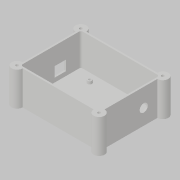
# Autodesk Inventor part: Pulsar_Box
Saved by Autodesk Inventor 2017.3 (Build 213256000, 256)
## iProperties
Created: 2018-02-02
Part Number: Pulsar_Box
Material: Generic
Document SubType Name: Modeling
Designer: Alex
Density: 1 g/cm^3
Appearance: Default
Author: Alex
Autodesk Inventor part; units mm, degrees
ref_plane "YZ Plane" through (0, 0, 0) normal (1, 0, 0) x (0, 1, 0)
ref_plane "XZ Plane" through (0, 0, 0) normal (0, 1, 0) x (-1, 0, 0)
ref_plane "XY Plane" through (0, 0, 0) normal (0, 0, 1) x (1, 0, 0)
sketch "Sketch1" plane through (0, 0, 0) normal (0, 1, 0) x (-1, 0, 0)
  line L0 (-45, 35) -> (-39, 35) construction
  line L1 (45, 35) -> (45, 29) construction
  line L2 (45, -35) -> (39, -35) construction
  line L3 (-45, -35) -> (-45, -29) construction
  line L4 (-45, 35) -> (45, -35) construction
  line L5 (45, 35) -> (-45, -35) construction
  arc A0 (40.2639, -31.3164) -> (39, -35) centre (45, -35) ccw construction
  arc A1 (-45, -29) -> (-39, -35) centre (-45, -35) ccw
  arc A2 (-40.2639, 31.3164) -> (-39, 35) centre (-45, 35) ccw construction
  arc A3 (45, 29) -> (39, 35) centre (45, 35) ccw
  line L6 (39, -35) -> (-39, -35)
  line L7 (45, -29) -> (45, -35) construction
  arc A4 (45, -29) -> (40.2639, -31.3164) centre (45, -35) ccw construction
  arc A5 (39, -35) -> (45, -29) centre (45, -35) ccw
  arc A6 (40.2639, 31.3164) -> (45, 29) centre (45, 35) ccw construction
  arc A7 (39, 35) -> (40.2639, 31.3164) centre (45, 35) ccw construction
  line L8 (39, 35) -> (45, 35) construction
  line L9 (45, 29) -> (45, -29)
  line L10 (-39, 35) -> (39, 35)
  line L11 (-45, 29) -> (-45, 35) construction
  arc A8 (-45, 29) -> (-40.2639, 31.3164) centre (-45, 35) ccw construction
  arc A9 (-39, 35) -> (-45, 29) centre (-45, 35) ccw
  arc A10 (-40.2639, -31.3164) -> (-45, -29) centre (-45, -35) ccw construction
  arc A11 (-39, -35) -> (-40.2639, -31.3164) centre (-45, -35) ccw construction
  line L12 (-39, -35) -> (-45, -35) construction
  line L13 (-45, -29) -> (-45, 29)
  point P0 (0, 0)
  dimension "d0" = 90
  dimension "d1" = 70
  dimension "d2" = 12
  constraints: 28 end point, 24 point on circle, 18 parallel, 12 centre point, 9 perpendicular, 4 coincident, 4 point on line, 3 equal radius, 3 horizontal, 2 midpoint
  measures "d0" distance of L2.start L3.start
  measures "d1" distance of L3.start L0.start
  measures "d2" diameter of A0
extrude "Extrusion1" add sketch "Sketch1" along normal blind 2
sketch "Sketch2" plane through (0, 2, 0) normal (0, 1, 0) x (1, 0, 0)
  line L0 (39, 35) -> (-39, 35) projected
  arc A0 (-39, 35) -> (-45, 29) centre (-45, 35) ccw projected
  line L1 (-45, 29) -> (-45, -29) projected
  arc A1 (-45, -29) -> (-39, -35) centre (-45, -35) ccw projected
  line L2 (-39, -35) -> (39, -35) projected
  arc A2 (39, -35) -> (45, -29) centre (45, -35) ccw projected
  line L3 (45, -29) -> (45, 29) projected
  arc A3 (45, 29) -> (39, 35) centre (45, 35) ccw projected
  line L4 (-41, 33) -> (41, 33)
  arc A4 (43, 31.5359) -> (41.5359, 33) centre (45, 35) ccw construction
  line L5 (43, 31) -> (43, -31)
  arc A5 (48.4641, -33) -> (43, -38.4641) centre (45, -35) ccw construction
  line L6 (41, -33) -> (-41, -33)
  arc A6 (-43, -31.5359) -> (-41.5359, -33) centre (-45, -35) ccw construction
  line L7 (-43, -31) -> (-43, 31)
  arc A7 (-48.4641, 33) -> (-43, 38.4641) centre (-45, 35) ccw construction
  arc A8 (-41, 33) -> (-43, 31) centre (-41, 31) ccw
  arc A9 (-43, -31) -> (-41, -33) centre (-41, -31) ccw
  arc A10 (41, -33) -> (43, -31) centre (41, -31) ccw
  arc A11 (43, 31) -> (41, 33) centre (41, 31) ccw
  point P0 (0, 0)
  dimension "d5" = 2
  dimension "d6" = 2
  constraints: 16 point on circle, 8 centre point, 8 end point, 8 point on line, 8 tangent, 3 equal radius, 7 other
  measures "d5" distance between parallel lines of L0 L4
  measures "d6" radius of A8
extrude "Extrusion2" add sketch "Sketch2" along normal blind 35
sketch "Sketch3" plane through (0, 2, 0) normal (0, 1, 0) x (1, 0, 0)
  arc A0 (-41, 33) -> (-43, 31) centre (-41, 31) ccw construction
  line L0 (-43, 31) -> (-43, -31) construction
  arc A1 (-43, -31) -> (-41, -33) centre (-41, -31) ccw construction
  line L1 (-41, -33) -> (41, -33) construction
  arc A2 (41, -33) -> (43, -31) centre (41, -31) ccw construction
  line L2 (43, -31) -> (43, 31) construction
  arc A3 (43, 31) -> (41, 33) centre (41, 31) ccw construction
  line L3 (41, 33) -> (-41, 33) construction
  arc A4 (-41, 33) -> (-43, 31) centre (-41, 31) ccw construction
  line L4 (-41, 33) -> (41, 33) construction
  arc A5 (43, 31) -> (41, 33) centre (41, 31) ccw construction
  line L5 (43, 31) -> (43, -31) construction
  arc A6 (41, -33) -> (43, -31) centre (41, -31) ccw construction
  line L6 (41, -33) -> (-41, -33) construction
  arc A7 (-43, -31) -> (-41, -33) centre (-41, -31) ccw construction
  line L7 (-43, -31) -> (-43, 31) construction
  line L8 (39, 35) -> (-39, 35) construction
  arc A8 (-39, 35) -> (-45, 29) centre (-45, 35) ccw construction
  line L9 (-45, 29) -> (-45, -29) construction
  arc A9 (-45, -29) -> (-39, -35) centre (-45, -35) ccw construction
  line L10 (-39, -35) -> (39, -35) construction
  arc A10 (39, -35) -> (45, -29) centre (45, -35) ccw construction
  line L11 (45, -29) -> (45, 29) construction
  arc A11 (45, 29) -> (39, 35) centre (45, 35) ccw construction
  circle A12 centre (-23.7, 23.4) radius 2.5
  circle A13 centre (27.1, 8.2) radius 2.5
  circle A14 centre (-25, -24.8) radius 2.5
  circle A15 centre (27.1, -19.7) radius 2.5
  line L12 (29.6, -27.3) -> (-39, -27.3) construction
  line L13 (-39, -27.3) -> (-39, 26) construction
  line L14 (-39, 26) -> (29.6, 26) construction
  line L15 (29.6, 26) -> (29.6, -27.3) construction
  line L16 (29.6, -27.3) -> (-39, 26) construction
  line L17 (-39, -27.3) -> (29.6, 26) construction
  circle A16 centre (-23.7, 23.4) radius 1.25
  circle A17 centre (27.1, 8.2) radius 1.25
  circle A18 centre (27.1, -19.7) radius 1.25
  circle A19 centre (-25, -24.8) radius 1.25
  point P0 (0, 0)
  point P1 (-4.7, -0.65)
  dimension "d9" = 5
  dimension "d10" = 53.3
  dimension "d11" = 68.6
  dimension "d12" = 2.5
  dimension "d13" = 5.1
  dimension "d14" = 27.9
  dimension "d15" = 15.2
  dimension "d16" = 14
  dimension "d17" = 1.3
  dimension "d18" = 50.8
  dimension "d19" = 4
  dimension "d20" = 7
  dimension "d21" = 2.5
  constraints: 12 end point, 8 centre point, 6 equal radius, 4 coincident, 2 midpoint, 2 parallel, 1 horizontal, 1 perpendicular, 1 vertical alignment
  measures "d9" diameter of A12
  measures "d10" distance of L12.end L13.end
  measures "d11" distance of L12.start L12.end
  measures "d12" distance from line of A14.centre L12
  measures "d13" vertical distance of A15.centre A14.centre
  measures "d14" distance of A13.centre A15.centre
  measures "d15" vertical distance of A12.centre A13.centre
  measures "d16" distance from line of L13 A14.centre
  measures "d17" horizontal distance of A12.centre A14.centre
  measures "d18" horizontal distance of A13.centre A12.centre
  measures "d19" distance between parallel lines of L0 L13
  measures "d20" distance between parallel lines of L4 L14
  measures "d21" diameter of A16
extrude "Extrusion3" add sketch "Sketch3" along normal blind 3
sketch "Sketch4" plane through (-43, 2, 31) normal (1, 0, 0) x (0, 0, -1)
  line L0 (62, 0) -> (0, 0) construction
  line L1 (62, 0) -> (62, 35) construction
  line L2 (0, 35) -> (62, 35) construction
  line L3 (0, 0) -> (0, 35) construction
  line L4 (2, -2) -> (60, -2) construction
  line L5 (2, -2) -> (2, 35) construction
  line L6 (60, 35) -> (2, 35) construction
  line L7 (60, -2) -> (60, 35) construction
  line L8 (8.7, 3) -> (3.7, 3) construction
  line L9 (3.7, 0) -> (8.7, 0) construction
  line L10 (3.7, 0) -> (3.7, 3) construction
  line L11 (8.7, 0) -> (8.7, 3) construction
  line L12 (4.95, 3) -> (7.45, 3) construction
  line L13 (7.45, 0) -> (4.95, 0) construction
  line L14 (4.95, 3) -> (7.45, 3) construction
  line L15 (7.45, 0) -> (7.45, 3) construction
  line L16 (4.95, 0) -> (4.95, 3) construction
  line L17 (56.9, 3) -> (51.9, 3) construction
  line L18 (51.9, 0) -> (56.9, 0) construction
  line L19 (56.9, 0) -> (56.9, 3) construction
  line L20 (51.9, 0) -> (51.9, 3) construction
  line L21 (53.15, 3) -> (55.65, 3) construction
  line L22 (53.15, 0) -> (53.15, 3) construction
  line L23 (55.65, 0) -> (55.65, 3) construction
  line L24 (0, 35) -> (62, 35) construction
  line L25 (47.7, 35) -> (47.7, 0) construction
  line L26 (62, 0) -> (0, 0) construction
  line L27 (35.2, 0) -> (35.2, 35) construction
  line L28 (54.4, -0.499) -> (54.4, 3) construction
  line L29 (35.2, 15.6) -> (47.7, 15.6)
  line L30 (47.7, 15.6) -> (47.7, 4.6)
  line L31 (47.7, 4.6) -> (35.2, 4.6)
  line L32 (35.2, 4.6) -> (35.2, 15.6)
  point P0 (31, -2)
  dimension "d25" = 6.7
  dimension "d26" = 12.5
  dimension "d27" = 11
  dimension "d28" = 1.6
  constraints: 14 end point, 4 point on line, 3 perpendicular, 2 parallel, 1 horizontal, 1 midpoint, 4 other
  measures "d25" distance between parallel lines of L25 L28
  measures "d26" distance between parallel lines of L27 L25
  measures "d27" distance between parallel lines of L31 L29
  measures "d28" distance between parallel lines of L31 L21
extrude "Extrusion4" cut sketch "Sketch4" against normal blind 3
sketch "Sketch5" plane through (45, 0, 29) normal (1, 0, 0) x (0, 0, -1)
  line L0 (58, 0) -> (0, 0) construction
  line L1 (58, 0) -> (58, 37) construction
  line L2 (0, 37) -> (58, 37) construction
  line L3 (0, 0) -> (0, 37) construction
  line L4 (33.2, 6.6) -> (33.2, 17.6) construction
  line L5 (33.2, 17.6) -> (45.7, 17.6) construction
  line L6 (45.7, 17.6) -> (45.7, 6.6) construction
  line L7 (45.7, 6.6) -> (33.2, 6.6) construction
  line L8 (60, 2) -> (-2, 2) construction
  line L9 (60, 2) -> (60, 37) construction
  line L10 (-2, 37) -> (60, 37) construction
  line L11 (-2, 2) -> (-2, 37) construction
  line L12 (33.2, 17.6) -> (45.7, 17.6) construction
  circle A0 centre (43, 17) radius 4.5
  line L13 (-2, 2) -> (60, 2) projected
  point P0 (29, 0)
  dimension "d31" = 9
  dimension "d32" = 15
  dimension "d33" = 15
  constraints: 1 centre point
  measures "d31" diameter of A0
  measures "d32" distance from line of L13 A0.centre
  measures "d33" distance from line of L1 A0.centre
extrude "Extrusion5" cut sketch "Sketch5" against normal blind 3
sketch "Sketch6" plane through (0, 37, 0) normal (0, 1, 0) x (1, 0, 0)
  arc A0 (-41, 33) -> (-43, 31) centre (-41, 31) ccw construction
  line L0 (-41, 33) -> (41, 33) construction
  arc A1 (43, 31) -> (41, 33) centre (41, 31) ccw construction
  line L1 (43, 31) -> (43, -31) construction
  arc A2 (41, -33) -> (43, -31) centre (41, -31) ccw construction
  line L2 (41, -33) -> (-41, -33) construction
  arc A3 (-43, -31) -> (-41, -33) centre (-41, -31) ccw construction
  line L3 (-43, -31) -> (-43, 31) construction
  line L4 (39, 35) -> (-39, 35) construction
  arc A4 (-39, 35) -> (-45, 29) centre (-45, 35) ccw construction
  line L5 (-45, 29) -> (-45, -29) construction
  arc A5 (-45, -29) -> (-39, -35) centre (-45, -35) ccw construction
  line L6 (-39, -35) -> (39, -35) construction
  arc A6 (39, -35) -> (45, -29) centre (45, -35) ccw construction
  line L7 (45, -29) -> (45, 29) construction
  arc A7 (45, 29) -> (39, 35) centre (45, 35) ccw construction
  arc A8 (39, -35) -> (45, -29) centre (45, -35) ccw projected
  point P0 (0, 0)
  constraints: 4 coincident
hole "Hole1" at (-45, 37, 35) at (-45, 37, -35) at (45, 37, -35) at (45, 37, 35) direction (0, -1, 0) diameter 3 depth 8 tip angle 118
sketch "Sketch7" plane through (39, 0, -35) normal (0, 0, -1) x (-1, 0, 0)
  line L0 (14, 28.5) -> (64, 28.5) construction
  line L1 (64, 28.5) -> (64, 8.5) construction
  line L2 (64, 8.5) -> (14, 8.5) construction
  line L3 (14, 8.5) -> (14, 28.5) construction
  line L4 (78, 0) -> (0, 0) construction
  line L5 (78, 0) -> (78, 37) construction
  line L6 (0, 37) -> (78, 37) construction
  line L7 (0, 0) -> (0, 37) construction
  spline S0 degree 2 poles (27.723, 19.9102) (27.723, 19.2121) (26.9874, 18.3594) (26.3034, 18.3594) knots 0 0 0 1 2 2 2
  line L8 (26.3034, 18.3594) -> (24.5746, 18.3594)
  line L9 (24.5746, 18.3594) -> (24.5746, 15.8108)
  spline S1 degree 2 poles (24.5746, 15.8108) (24.5746, 15.4313) (24.2185, 15.4313) knots 0 0 0 1 1 1
  spline S2 degree 2 poles (24.2185, 15.4313) (23.8578, 15.4313) (23.8578, 15.8108) knots 0 0 0 1 1 1
  line L10 (23.8578, 15.8108) -> (23.8578, 21.5219)
  line L11 (23.8578, 21.5219) -> (26.1628, 21.5219)
  spline S3 degree 2 poles (26.1628, 21.5219) (26.9593, 21.5219) (27.3575, 21.0627) knots 0 0 0 1 1 1
  spline S4 degree 2 poles (27.3575, 21.0627) (27.723, 20.6458) (27.723, 19.9102) knots 0 0 0 1 1 1
  spline S5 degree 2 poles (27.0061, 19.9102) (27.0061, 20.7863) (26.1628, 20.7863) knots 0 0 0 1 1 1
  line L12 (26.1628, 20.7863) -> (24.5746, 20.7863)
  line L13 (24.5746, 20.7863) -> (24.5746, 19.1044)
  line L14 (24.5746, 19.1044) -> (26.3034, 19.1044)
  spline S6 degree 2 poles (26.3034, 19.1044) (27.0061, 19.1044) (27.0061, 19.9102) knots 0 0 0 1 1 1
  spline S7 degree 2 poles (32.9796, 17.4693) (32.9796, 15.5437) (30.9838, 15.3938) knots 0 0 0 1 1 1
  spline S8 degree 2 poles (30.9838, 15.3938) (30.1498, 15.3329) (29.4939, 15.8482) knots 0 0 0 1 1 1
  spline S9 degree 2 poles (29.4939, 15.8482) (28.7677, 16.4245) (28.7677, 17.4177) knots 0 0 0 1 1 1
  line L15 (28.7677, 17.4177) -> (28.7677, 21.1518)
  spline S10 degree 2 poles (28.7677, 21.1518) (28.7677, 21.5313) (29.1332, 21.5313) knots 0 0 0 1 1 1
  spline S11 degree 2 poles (29.1332, 21.5313) (29.4939, 21.5313) (29.4939, 21.1518) knots 0 0 0 1 1 1
  line L16 (29.4939, 21.1518) -> (29.4939, 17.4177)
  spline S12 degree 2 poles (29.4939, 17.4177) (29.4939, 16.7759) (29.9624, 16.4151) knots 0 0 0 1 1 1
  spline S13 degree 2 poles (29.9624, 16.4151) (30.3794, 16.0919) (30.9323, 16.1293) knots 0 0 0 1 1 1
  spline S14 degree 2 poles (30.9323, 16.1293) (32.2628, 16.209) (32.2628, 17.4693) knots 0 0 0 1 1 1
  line L17 (32.2628, 17.4693) -> (32.2628, 21.1518)
  spline S15 degree 2 poles (32.2628, 21.1518) (32.2628, 21.5313) (32.6236, 21.5313) knots 0 0 0 1 1 1
  spline S16 degree 2 poles (32.6236, 21.5313) (32.9796, 21.5313) (32.9796, 21.1518) knots 0 0 0 1 1 1
  line L18 (32.9796, 21.1518) -> (32.9796, 17.4693)
  line L19 (37.646, 15.5109) -> (34.0197, 15.5109)
  line L20 (34.0197, 15.5109) -> (34.0197, 21.1424)
  spline S17 degree 2 poles (34.0197, 21.1424) (34.0197, 21.5219) (34.3805, 21.5219) knots 0 0 0 1 1 1
  spline S18 degree 2 poles (34.3805, 21.5219) (34.7366, 21.5219) (34.7366, 21.1424) knots 0 0 0 1 1 1
  line L21 (34.7366, 21.1424) -> (34.7366, 16.2465)
  line L22 (34.7366, 16.2465) -> (37.646, 16.2465)
  spline S19 degree 2 poles (37.646, 16.2465) (38.0114, 16.2465) (38.0114, 15.881) knots 0 0 0 1 1 1
  spline S20 degree 2 poles (38.0114, 15.881) (38.0114, 15.5109) (37.646, 15.5109) knots 0 0 0 1 1 1
  spline S21 degree 2 poles (43.0995, 17.1132) (43.0995, 15.3938) (40.9537, 15.3938) knots 0 0 0 1 1 1
  spline S22 degree 2 poles (40.9537, 15.3938) (39.6653, 15.3938) (38.9719, 16.6728) knots 0 0 0 1 1 1
  spline S23 degree 2 poles (38.9719, 16.6728) (38.9204, 16.7618) (38.9204, 16.8696) knots 0 0 0 1 1 1
  spline S24 degree 2 poles (38.9204, 16.8696) (38.9204, 17.0382) (39.1687, 17.2959) (39.3186, 17.2959) knots 0 0 0 1 2 2 2
  spline S25 degree 2 poles (39.3186, 17.2959) (39.4872, 17.2959) (39.5669, 17.1085) knots 0 0 0 1 1 1
  spline S26 degree 2 poles (39.5669, 17.1085) (40.0026, 16.1387) (40.9537, 16.1387) knots 0 0 0 1 1 1
  spline S27 degree 2 poles (40.9537, 16.1387) (42.3545, 16.1387) (42.3545, 17.1038) knots 0 0 0 1 1 1
  spline S28 degree 2 poles (42.3545, 17.1038) (42.3545, 17.6005) (41.4737, 17.9659) knots 0 0 0 1 1 1
  spline S29 degree 2 poles (41.4737, 17.9659) (39.8855, 18.6312) (39.8527, 18.6499) knots 0 0 0 1 1 1
  spline S30 degree 2 poles (39.8527, 18.6499) (38.9719, 19.1747) (38.9719, 20.0414) knots 0 0 0 1 1 1
  spline S31 degree 2 poles (38.9719, 20.0414) (38.9719, 20.8566) (39.5669, 21.2736) knots 0 0 0 1 1 1
  spline S32 degree 2 poles (39.5669, 21.2736) (40.0448, 21.6109) (40.8272, 21.639) knots 0 0 0 1 1 1
  spline S33 degree 2 poles (40.8272, 21.639) (41.544, 21.6671) (42.0781, 21.3485) knots 0 0 0 1 1 1
  spline S34 degree 2 poles (42.0781, 21.3485) (42.645, 21.0018) (42.8512, 20.3553) knots 0 0 0 1 1 1
  spline S35 degree 2 poles (42.8512, 20.3553) (42.8652, 20.2897) (42.8652, 20.2288) knots 0 0 0 1 1 1
  spline S36 degree 2 poles (42.8652, 20.2288) (42.8652, 20.0789) (42.645, 19.8915) (42.4951, 19.8915) knots 0 0 0 1 2 2 2
  spline S37 degree 2 poles (42.4951, 19.8915) (42.228, 19.8915) (42.1484, 20.1492) knots 0 0 0 1 1 1
  spline S38 degree 2 poles (42.1484, 20.1492) (42.0313, 20.5146) (41.2957, 20.9316) (40.8506, 20.9128) knots 0 0 0 1 2 2 2
  spline S39 degree 2 poles (40.8506, 20.9128) (39.6887, 20.8707) (39.6887, 20.0601) knots 0 0 0 1 1 1
  spline S40 degree 2 poles (39.6887, 20.0601) (39.6887, 19.6432) (40.1057, 19.3527) knots 0 0 0 1 1 1
  spline S41 degree 2 poles (40.1057, 19.3527) (40.4008, 19.1465) (41.0849, 18.8982) knots 0 0 0 1 1 1
  spline S42 degree 2 poles (41.0849, 18.8982) (42.0969, 18.5328) (42.4435, 18.2939) knots 0 0 0 1 1 1
  spline S43 degree 2 poles (42.4435, 18.2939) (43.0995, 17.8441) (43.0995, 17.1132) knots 0 0 0 1 1 1
  spline S44 degree 2 poles (48.8996, 15.9279) (48.923, 15.8482) (48.923, 15.778) knots 0 0 0 1 1 1
  spline S45 degree 2 poles (48.923, 15.778) (48.923, 15.628) (48.6935, 15.4313) (48.5529, 15.4313) knots 0 0 0 1 2 2 2
  spline S46 degree 2 poles (48.5529, 15.4313) (48.2999, 15.4313) (48.2109, 15.6608) knots 0 0 0 1 1 1
  line L23 (48.2109, 15.6608) -> (47.8595, 16.5651)
  line L24 (47.8595, 16.5651) -> (44.9594, 16.5651)
  line L25 (44.9594, 16.5651) -> (44.6127, 15.6608)
  spline S47 degree 2 poles (44.6127, 15.6608) (44.5237, 15.4313) (44.2848, 15.4313) knots 0 0 0 1 1 1
  spline S48 degree 2 poles (44.2848, 15.4313) (44.1349, 15.4313) (43.9053, 15.6327) (43.9053, 15.778) knots 0 0 0 1 2 2 2
  spline S49 degree 2 poles (43.9053, 15.778) (43.9053, 15.8482) (43.9334, 15.9279) knots 0 0 0 1 1 1
  line L26 (43.9334, 15.9279) -> (45.9339, 21.2923)
  spline S50 degree 2 poles (45.9339, 21.2923) (46.0417, 21.5781) (46.3697, 21.5781) knots 0 0 0 1 1 1
  spline S51 degree 2 poles (46.3697, 21.5781) (46.707, 21.5781) (46.8147, 21.2923) knots 0 0 0 1 1 1
  line L27 (46.8147, 21.2923) -> (48.8996, 15.9279)
  line L28 (47.5831, 17.31) -> (46.3697, 20.4115)
  line L29 (46.3697, 20.4115) -> (45.2406, 17.31)
  line L30 (45.2406, 17.31) -> (47.5831, 17.31)
  spline S52 degree 2 poles (54.0251, 19.7697) (54.0251, 18.8467) (53.4207, 18.3829) knots 0 0 0 1 1 1
  spline S53 degree 2 poles (53.4207, 18.3829) (53.0225, 18.083) (52.6243, 18.083) knots 0 0 0 1 1 1
  line L31 (52.6243, 18.083) -> (52.5353, 18.0783)
  line L32 (52.5353, 18.0783) -> (53.9548, 16.045)
  spline S54 degree 2 poles (53.9548, 16.045) (54.0251, 15.9373) (54.0251, 15.8201) knots 0 0 0 1 1 1
  spline S55 degree 2 poles (54.0251, 15.8201) (54.0251, 15.6702) (53.7955, 15.4406) (53.655, 15.4406) knots 0 0 0 1 2 2 2
  spline S56 degree 2 poles (53.655, 15.4406) (53.4863, 15.4406) (53.3786, 15.5999) knots 0 0 0 1 1 1
  line L33 (53.3786, 15.5999) -> (51.631, 18.083)
  line L34 (51.631, 18.083) -> (50.4691, 18.083)
  line L35 (50.4691, 18.083) -> (50.4691, 15.8201)
  spline S57 degree 2 poles (50.4691, 15.8201) (50.4691, 15.4406) (50.1084, 15.4406) knots 0 0 0 1 1 1
  spline S58 degree 2 poles (50.1084, 15.4406) (49.7429, 15.4406) (49.7429, 15.8201) knots 0 0 0 1 1 1
  line L36 (49.7429, 15.8201) -> (49.7429, 21.5172)
  line L37 (49.7429, 21.5172) -> (52.3057, 21.5172)
  spline S59 degree 2 poles (52.3057, 21.5172) (53.0038, 21.5172) (53.5004, 21.0627) knots 0 0 0 1 1 1
  spline S60 degree 2 poles (53.5004, 21.0627) (54.0251, 20.5661) (54.0251, 19.7697) knots 0 0 0 1 1 1
  spline S61 degree 2 poles (53.3083, 19.7697) (53.3083, 20.2382) (53.0084, 20.524) knots 0 0 0 1 1 1
  spline S62 degree 2 poles (53.0084, 20.524) (52.7227, 20.7816) (52.3057, 20.7816) knots 0 0 0 1 1 1
  line L38 (52.3057, 20.7816) -> (50.4691, 20.7816)
  line L39 (50.4691, 20.7816) -> (50.4691, 18.828)
  line L40 (50.4691, 18.828) -> (52.6243, 18.828)
  spline S63 degree 2 poles (52.6243, 18.828) (52.821, 18.828) (53.0225, 19.0154) knots 0 0 0 1 1 1
  spline S64 degree 2 poles (53.0225, 19.0154) (53.3083, 19.273) (53.3083, 19.7697) knots 0 0 0 1 1 1
  point P0 (39, 0)
  point P1 (39, 37)
  point P2 (39, 28.5)
  point P3 (14, 18.5)
  point P4 (0, 18.5)
  point P5 (64, 18.5)
  dimension "d43" = 50
  dimension "d44" = 20
  constraints: 5 midpoint, 2 horizontal alignment, 1 vertical alignment, 2 other
  measures "d43" distance of L1.end L2.end
  measures "d44" distance of L0.end L1.end
emboss "Emboss1" sketch "Sketch7" operation add depth 1 direction (0, 0, 1)
body "Solid1"
